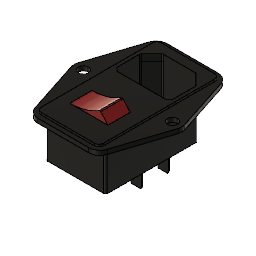
Controller PSU Assembly (Autodesk Fusion 360 archive; units mm, degrees)
design "IEC Inlet"
Autodesk Fusion 360 part; units mm, degrees
sketch "Sketch1" plane through (0, 0, 0) normal (0, 0, 1) x (1, 0, 0)
  line L0 (-25, 14) -> (25, 14)
  line L1 (27, 12) -> (27, -12)
  line L2 (25, -14) -> (-25, -14)
  line L3 (-27, -12) -> (-27, 12)
  arc A0 (-25, 14) -> (-27, 12) centre (-25, 12) ccw
  arc A1 (-27, -12) -> (-25, -14) centre (-25, -12) ccw
  arc A2 (25, -14) -> (27, -12) centre (25, -12) ccw
  arc A3 (27, 12) -> (25, 14) centre (25, 12) ccw
  dimension "d1" = 28
  dimension "d2" = 54
  dimension "d3" = 14
  dimension "d4" = 27
  dimension "d5" = 2
  constraint horizontal L0
  constraint vertical L1
  constraint horizontal L2
  constraint vertical L3
  constraint tangent L3 A0
  constraint tangent L0 A0
  constraint tangent L3 A1
  constraint tangent L2 A1
  constraint equal A0 A1
  constraint tangent L2 A2
  constraint tangent L1 A2
  constraint equal A0 A2
  constraint tangent L1 A3
  constraint tangent L0 A3
  constraint equal A0 A3
  measures "d1" distance of L0 L2
  measures "d2" distance of L1 L3
  measures "d3" distance of origin L2
  measures "d4" distance of origin L3
  measures "d5" radius of A0
extrude "Extrude1" add sketch "Sketch1" along normal blind 1
sketch "Sketch2" plane through (0, 0, 0) normal (0, 0, -1) x (1, 0, 0)
  arc A0 (27, 12) -> (25, 14) centre (25, 12) ccw
  line L0 (25, 14) -> (-25, 14)
  arc A1 (-25, 14) -> (-27, 12) centre (-25, 12) ccw
  line L1 (-27, 12) -> (-27, -12)
  arc A2 (-27, -12) -> (-25, -14) centre (-25, -12) ccw
  line L2 (-25, -14) -> (25, -14)
  arc A3 (25, -14) -> (27, -12) centre (25, -12) ccw
  line L3 (27, -12) -> (27, 12)
  line L4 (-29, 24.5) -> (29, 24.5)
  line L5 (29, 11.423) -> (29, -11.423)
  line L6 (29, -24.5) -> (-29, -24.5)
  line L7 (-29, -11.423) -> (-29, 11.423)
  circle A4 centre (0, -20) radius 2.25
  circle A5 centre (0, 20) radius 2.25
  line L8 (1.5487, -23.9955) -> (25.5487, -16.1771)
  line L9 (-1.5487, -23.9955) -> (-25.5487, -16.1771)
  line L10 (1.5487, 23.9955) -> (25.5487, 16.1771)
  line L11 (-1.5487, 23.9955) -> (-25.5487, 16.1771)
  arc A6 (25.5487, -16.1771) -> (29, -11.423) centre (24, -11.423) ccw
  arc A7 (29, 11.423) -> (25.5487, 16.1771) centre (24, 11.423) ccw
  arc A8 (-25.5487, 16.1771) -> (-29, 11.423) centre (-24, 11.423) ccw
  arc A9 (-29, -11.423) -> (-25.5487, -16.1771) centre (-24, -11.423) ccw
  arc A10 (-1.5487, -23.9955) -> (1.5487, -23.9955) centre (0, -19.2414) ccw
  arc A11 (1.5487, 23.9955) -> (-1.5487, 23.9955) centre (0, 19.2414) ccw
  point P0 (0, -24.5)
  point P1 (29, -15.0528)
  point P2 (-29, -15.0528)
  point P3 (0, 24.5)
  point P4 (29, 15.0528)
  point P5 (-29, 15.0528)
  dimension "d8" = 58
  dimension "d9" = 29
  dimension "d10" = 49
  dimension "d11" = 24.5
  dimension "d12" = 4.5
  dimension "d13" = 4.5
  dimension "d14" = 40
  dimension "d15" = 4.5
  dimension "d16" = 30.5
  dimension "d17" = 30.5
  dimension "d18" = 30.5
  dimension "d19" = 30.5
  dimension "d20" = 5
  dimension "d21" = 5
  constraint horizontal L4
  constraint vertical L5
  constraint horizontal L6
  constraint vertical L7
  constraint vertical origin A5.centre
  constraint vertical origin A4.centre
  constraint midpoint L6 P0
  constraint coincident L5 P1
  constraint coincident L7 P2
  constraint midpoint L4 P3
  constraint coincident L5 P4
  constraint coincident L7 P5
  constraint coincident P1 L8
  constraint coincident L6.start L5
  constraint tangent L8 A6
  constraint tangent L5 A6
  constraint coincident L4.end L5
  constraint coincident P4 L10
  constraint tangent L5 A7
  constraint tangent L10 A7
  constraint equal A6 A7
  constraint coincident P5 L11
  constraint coincident L4.start L7
  constraint tangent L11 A8
  constraint tangent L7 A8
  constraint equal A6 A8
  constraint coincident L6.end L7
  constraint coincident P2 L9
  constraint tangent L7 A9
  constraint tangent L9 A9
  constraint equal A6 A9
  constraint coincident P0 L9
  constraint coincident P0 L8
  constraint tangent L9 A10
  constraint tangent L8 A10
  constraint coincident P3 L10
  constraint coincident P3 L11
  constraint tangent L10 A11
  constraint tangent L11 A11
  constraint equal A10 A11
  measures "d8" distance of L5 L7
  measures "d9" distance of origin L7
  measures "d10" distance of L4 L6
  measures "d11" distance of origin L6
  measures "d12" diameter of A4
  measures "d13" diameter of A5
  measures "d14" distance of A4.centre A5.centre
  measures "d15" distance of L6 A4.centre
  measures "d16" distance of P0 P1
  measures "d17" distance of P0 P2
  measures "d18" distance of P3 P4
  measures "d19" distance of P3 P5
  measures "d20" radius of A6
  measures "d21" radius of A10
extrude "Extrude2" add sketch "Sketch2" along normal blind 2 contours A0 L0 A1 L1 A2 L2 A3 L3 | L5 L7 L8 L9 L10 L11 A6 A7 A8 A9 A10 A11
sketch "Sketch3" plane through (0, 0, -2) normal (0, 0, -1) x (1, 0, 0)
  circle A0 centre (0, 20) radius 2.25
  circle A1 centre (0, -20) radius 2.25
  arc A2 (29, 11.423) -> (25.5487, 16.1771) centre (24, 11.423) ccw
  line L0 (25.5487, 16.1771) -> (1.5487, 23.9955)
  arc A3 (1.5487, 23.9955) -> (-1.5487, 23.9955) centre (0, 19.2414) ccw
  line L1 (-1.5487, 23.9955) -> (-25.5487, 16.1771)
  arc A4 (-25.5487, 16.1771) -> (-29, 11.423) centre (-24, 11.423) ccw
  line L2 (-29, 11.423) -> (-29, -11.423)
  arc A5 (-29, -11.423) -> (-25.5487, -16.1771) centre (-24, -11.423) ccw
  line L3 (-25.5487, -16.1771) -> (-1.5487, -23.9955)
  arc A6 (-1.5487, -23.9955) -> (1.5487, -23.9955) centre (0, -19.2414) ccw
  line L4 (1.5487, -23.9955) -> (25.5487, -16.1771)
  arc A7 (25.5487, -16.1771) -> (29, -11.423) centre (24, -11.423) ccw
  line L5 (29, -11.423) -> (29, 11.423)
  line L6 (-22.5, 13.5) -> (22.5, 13.5)
  line L7 (23.5, 12.5) -> (23.5, -12.5)
  line L8 (22.5, -13.5) -> (-22.5, -13.5)
  line L9 (-23.5, -12.5) -> (-23.5, 12.5)
  arc A8 (23.5, 12.5) -> (22.5, 13.5) centre (22.5, 12.5) ccw
  arc A9 (22.5, -13.5) -> (23.5, -12.5) centre (22.5, -12.5) ccw
  arc A10 (-23.5, -12.5) -> (-22.5, -13.5) centre (-22.5, -12.5) ccw
  arc A11 (-22.5, 13.5) -> (-23.5, 12.5) centre (-22.5, 12.5) ccw
  dimension "d24" = 27
  dimension "d25" = 47
  dimension "d26" = 23.5
  dimension "d27" = 13.5
  dimension "d30" = 1
  constraint horizontal L6
  constraint vertical L7
  constraint horizontal L8
  constraint vertical L9
  constraint tangent L6 A8
  constraint tangent L7 A8
  constraint tangent L7 A9
  constraint tangent L8 A9
  constraint equal A8 A9
  constraint tangent L8 A10
  constraint tangent L9 A10
  constraint equal A8 A10
  constraint tangent L9 A11
  constraint tangent L6 A11
  constraint equal A8 A11
  measures "d24" distance of L6 L8
  measures "d25" distance of L7 L9
  measures "d26" distance of origin L9
  measures "d27" distance of origin L6
  measures "d30" radius of A8
extrude "Extrude3" add sketch "Sketch3" along normal blind 18 contours L6 L7 L8 L9 A8 A9 A10 A11
sketch "Sketch4" plane through (0, 0, -20) normal (0, 0, -1) x (1, 0, 0)
  arc A0 (23.5, 12.5) -> (22.5, 13.5) centre (22.5, 12.5) ccw
  line L0 (22.5, 13.5) -> (-22.5, 13.5)
  arc A1 (-22.5, 13.5) -> (-23.5, 12.5) centre (-22.5, 12.5) ccw
  line L1 (-23.5, 12.5) -> (-23.5, -12.5)
  arc A2 (-23.5, -12.5) -> (-22.5, -13.5) centre (-22.5, -12.5) ccw
  line L2 (-22.5, -13.5) -> (22.5, -13.5)
  arc A3 (22.5, -13.5) -> (23.5, -12.5) centre (22.5, -12.5) ccw
  line L3 (23.5, -12.5) -> (23.5, 12.5)
  line L4 (17.136, 13.5) -> (23.5, 7.136)
  line L5 (23.5, -7.136) -> (17.136, -13.5)
  dimension "d31" = 9
  dimension "d32" = 9
  dimension "d33" = 45
  dimension "d34" = 45
  constraint coincident L0 L4.start
  constraint coincident L3 L4.end
  constraint coincident L3 L5.start
  constraint coincident L2 L5.end
  measures "d31" distance of L5.start L5.end
  measures "d32" distance of L4.start L4.end
  measures "d33" angle of L3 L4
  measures "d34" angle of L3 L5
extrude "Extrude4" cut sketch "Sketch4" against normal blind 18 contours A0 L0 L3 L4 | L2 A3 L3 L5
sketch "Sketch5" plane through (0, 0, 1) normal (0, 0, 1) x (-1, 0, 0)
  arc A0 (-25, 14) -> (-27, 12) centre (-25, 12) ccw
  line L0 (-27, 12) -> (-27, -12)
  arc A1 (-27, -12) -> (-25, -14) centre (-25, -12) ccw
  line L1 (-25, -14) -> (25, -14)
  arc A2 (25, -14) -> (27, -12) centre (25, -12) ccw
  line L2 (27, -12) -> (27, 12)
  arc A3 (27, 12) -> (25, 14) centre (25, 12) ccw
  line L3 (25, 14) -> (-25, 14)
  line L4 (-8, -12.5) -> (-17.636, -12.5)
  line L5 (-23, -7.136) -> (-23, 7.136)
  line L6 (-17.636, 12.5) -> (-8, 12.5)
  line L7 (-6, 10.5) -> (-6, -10.5)
  line L8 (-18.3431, 12.2071) -> (-22.7071, 7.8431)
  line L9 (-22.7071, -7.8431) -> (-18.3431, -12.2071)
  arc A4 (-8, -12.5) -> (-6, -10.5) centre (-8, -10.5) ccw
  arc A5 (-6, 10.5) -> (-8, 12.5) centre (-8, 10.5) ccw
  arc A6 (-18.3431, -12.2071) -> (-17.636, -12.5) centre (-17.636, -11.5) ccw
  arc A7 (-23, -7.136) -> (-22.7071, -7.8431) centre (-22, -7.136) ccw
  arc A8 (-22.7071, 7.8431) -> (-23, 7.136) centre (-22, 7.136) ccw
  arc A9 (-17.636, 12.5) -> (-18.3431, 12.2071) centre (-17.636, 11.5) ccw
  point P0 (-18.0503, 12.5)
  point P1 (-23, 7.5503)
  point P2 (-23, -7.5503)
  point P3 (-18.0503, -12.5)
  dimension "d37" = 4
  dimension "d38" = 17
  dimension "d39" = 25
  dimension "d40" = 12.5
  dimension "d41" = 7
  dimension "d42" = 7
  dimension "d43" = 45
  dimension "d44" = 45
  dimension "d45" = 2
  dimension "d46" = 1
  constraint horizontal L4
  constraint vertical L5
  constraint horizontal L6
  constraint vertical L7
  constraint coincident L6 P0
  constraint coincident L5 P1
  constraint coincident L5 P2
  constraint coincident L4 P3
  constraint tangent L4 A4
  constraint tangent L7 A4
  constraint tangent L6 A5
  constraint tangent L7 A5
  constraint equal A4 A5
  constraint coincident P3 L9
  constraint tangent L4 A6
  constraint tangent L9 A6
  constraint coincident P2 L9
  constraint tangent L9 A7
  constraint tangent L5 A7
  constraint equal A6 A7
  constraint coincident P1 L8
  constraint tangent L5 A8
  constraint tangent L8 A8
  constraint equal A6 A8
  constraint coincident P0 L8
  constraint tangent L8 A9
  constraint tangent L6 A9
  constraint equal A6 A9
  measures "d37" distance of L0 L5
  measures "d38" distance of L5 L7
  measures "d39" distance of L4 L6
  measures "d40" distance of origin L6
  measures "d41" distance of P0 P1
  measures "d42" distance of P2 P3
  measures "d43" angle of L5 L9
  measures "d44" angle of L5 L8
  measures "d45" radius of A4
  measures "d46" radius of A6
extrude "Extrude5" cut sketch "Sketch5" against normal blind 18 contours L4 L5 L6 L7 L8 L9 A4 A5 A6 A7 A8 A9
sketch "Sketch6" plane through (0, 0, 1) normal (0, 0, 1) x (-1, 0, 0)
  line L0 (-17.636, 12.5) -> (-8, 12.5)
  arc A0 (-6, 10.5) -> (-8, 12.5) centre (-8, 10.5) ccw
  line L1 (-6, 10.5) -> (-6, -10.5)
  arc A1 (-8, -12.5) -> (-6, -10.5) centre (-8, -10.5) ccw
  line L2 (-8, -12.5) -> (-17.636, -12.5)
  arc A2 (-18.3431, -12.2071) -> (-17.636, -12.5) centre (-17.636, -11.5) ccw
  line L3 (-18.3431, -12.2071) -> (-22.7071, -7.8431)
  arc A3 (-23, -7.136) -> (-22.7071, -7.8431) centre (-22, -7.136) ccw
  line L4 (-23, -7.136) -> (-23, 7.136)
  arc A4 (-22.7071, 7.8431) -> (-23, 7.136) centre (-22, 7.136) ccw
  line L5 (-22.7071, 7.8431) -> (-18.3431, 12.2071)
  arc A5 (-17.636, 12.5) -> (-18.3431, 12.2071) centre (-17.636, 11.5) ccw
  arc A6 (-25, 14) -> (-27, 12) centre (-25, 12) ccw
  line L6 (-27, 12) -> (-27, -12)
  arc A7 (-27, -12) -> (-25, -14) centre (-25, -12) ccw
  line L7 (-25, -14) -> (25, -14)
  arc A8 (25, -14) -> (27, -12) centre (25, -12) ccw
  line L8 (27, -12) -> (27, 12)
  arc A9 (27, 12) -> (25, 14) centre (25, 12) ccw
  line L9 (25, 14) -> (-25, 14)
  line L10 (17, -8) -> (7, -8)
  line L11 (7, -8) -> (7, 8)
  line L12 (7, 8) -> (17, 8)
  line L13 (17, 8) -> (17, -8)
  line L14 (17, 4.5) -> (7, 4.5)
  dimension "d49" = 16
  dimension "d50" = 10
  dimension "d51" = 10
  dimension "d52" = 6
  dimension "d53" = 12.5
  constraint horizontal L10
  constraint vertical L11
  constraint horizontal L12
  constraint vertical L13
  constraint coincident L13 L14.start
  constraint coincident L11 L14.end
  constraint perpendicular L11 L14
  measures "d49" distance of L10 L12
  measures "d50" distance of L11 L13
  measures "d51" distance of L8 L13
  measures "d52" distance of L7 L10
  measures "d53" distance of L10 L14
extrude "Extrude6" add sketch "Sketch6" along normal blind 4 contours L11 L12 L13 L14
fillet "Fillet1" radius 25 1 edges at (-12, -4.5, 1)
sketch "Sketch7" plane through (-17, 0, 0) normal (-1, 0, 0) x (0, -1, 0)
  line L0 (-9.0647, 1) -> (8, 1)
  line L1 (8, 1) -> (8, 5)
  line L2 (8, 5) -> (4.5, 5)
  arc A0 (-9.0647, 1) -> (4.5, 5) centre (-9.0647, 26) ccw
  line L3 (4.5, 5) -> (8, 1)
  constraint coincident L2.end A0.end
  constraint coincident L0.end L1.start
extrude "Extrude7" cut sketch "Sketch7" against normal blind 10 contours L1 L2 L3
fillet "Fillet2" radius 0.5 1 edges at (-12, -4.5, 5)
sketch "Sketch9" plane through (0, 0, -20) normal (0, 0, -1) x (1, 0, 0)
  line L0 (23.5, 7.136) -> (17.136, 13.5)
  line L1 (17.136, 13.5) -> (-22.5, 13.5)
  arc A0 (-22.5, 13.5) -> (-23.5, 12.5) centre (-22.5, 12.5) ccw
  line L2 (-23.5, 12.5) -> (-23.5, -12.5)
  arc A1 (-23.5, -12.5) -> (-22.5, -13.5) centre (-22.5, -12.5) ccw
  line L3 (-22.5, -13.5) -> (17.136, -13.5)
  line L4 (17.136, -13.5) -> (23.5, -7.136)
  line L5 (23.5, -7.136) -> (23.5, 7.136)
  line L6 (-21.5, 12.5) -> (-8.5, 12.5)
  line L7 (-7.5, 11.5) -> (-7.5, -11.5)
  line L8 (-8.5, -12.5) -> (-21.5, -12.5)
  line L9 (-22.5, -11.5) -> (-22.5, 11.5)
  arc A2 (-21.5, 12.5) -> (-22.5, 11.5) centre (-21.5, 11.5) ccw
  arc A3 (-7.5, 11.5) -> (-8.5, 12.5) centre (-8.5, 11.5) ccw
  arc A4 (-8.5, -12.5) -> (-7.5, -11.5) centre (-8.5, -11.5) ccw
  arc A5 (-22.5, -11.5) -> (-21.5, -12.5) centre (-21.5, -11.5) ccw
  dimension "d62" = 1
  dimension "d63" = 1
  dimension "d64" = 1
  dimension "d65" = 15
  dimension "d66" = 1
  constraint horizontal L6
  constraint vertical L7
  constraint horizontal L8
  constraint vertical L9
  constraint tangent L6 A2
  constraint tangent L9 A2
  constraint tangent L6 A3
  constraint tangent L7 A3
  constraint equal A2 A3
  constraint tangent L7 A4
  constraint tangent L8 A4
  constraint equal A2 A4
  constraint tangent L8 A5
  constraint tangent L9 A5
  constraint equal A2 A5
  measures "d62" distance of L1 L6
  measures "d63" distance of L3 L8
  measures "d64" distance of L2 L9
  measures "d65" distance of L7 L9
  measures "d66" radius of A2
extrude "Extrude8" cut sketch "Sketch9" against normal blind 18 contours L6 L7 L8 L9 A2 A3 A4 A5
sketch "Sketch10" plane through (0, 0, -20) normal (0, 0, -1) x (1, 0, 0)
  line L0 (-22.5, -11.5) -> (-22.5, 11.5)
  arc A0 (-21.5, 12.5) -> (-22.5, 11.5) centre (-21.5, 11.5) ccw
  line L1 (-21.5, 12.5) -> (-8.5, 12.5)
  arc A1 (-7.5, 11.5) -> (-8.5, 12.5) centre (-8.5, 11.5) ccw
  line L2 (-7.5, 11.5) -> (-7.5, -11.5)
  arc A2 (-8.5, -12.5) -> (-7.5, -11.5) centre (-8.5, -11.5) ccw
  line L3 (-8.5, -12.5) -> (-21.5, -12.5)
  arc A3 (-22.5, -11.5) -> (-21.5, -12.5) centre (-21.5, -11.5) ccw
  line L4 (23.5, 7.136) -> (17.136, 13.5)
  line L5 (17.136, 13.5) -> (-22.5, 13.5)
  arc A4 (-22.5, 13.5) -> (-23.5, 12.5) centre (-22.5, 12.5) ccw
  line L6 (-23.5, 12.5) -> (-23.5, -12.5)
  arc A5 (-23.5, -12.5) -> (-22.5, -13.5) centre (-22.5, -12.5) ccw
  line L7 (-22.5, -13.5) -> (17.136, -13.5)
  line L8 (17.136, -13.5) -> (23.5, -7.136)
  line L9 (23.5, -7.136) -> (23.5, 7.136)
  line L10 (19.5, 2.5) -> (20, 2.5)
  line L11 (20, 2.5) -> (20, -2.5)
  line L12 (20, -2.5) -> (19.5, -2.5)
  line L13 (19.5, -2.5) -> (19.5, 2.5)
  line L14 (8.636, 9.5) -> (9.136, 9.5)
  line L15 (9.136, 9.5) -> (9.136, 4.5)
  line L16 (9.136, 4.5) -> (8.636, 4.5)
  line L17 (8.636, 4.5) -> (8.636, 9.5)
  line L18 (-3.364, 9.5) -> (-2.864, 9.5)
  line L19 (-2.864, 9.5) -> (-2.864, 4.5)
  line L20 (-2.864, 4.5) -> (-3.364, 4.5)
  line L21 (-3.364, 4.5) -> (-3.364, 9.5)
  dimension "d69" = 5
  dimension "d70" = 0.5
  dimension "d71" = 0.5
  dimension "d72" = 5
  dimension "d75" = 3.5
  dimension "d76" = 11
  dimension "d77" = 4
  dimension "d78" = 5
  dimension "d79" = 0.5
  dimension "d80" = 4
  dimension "d81" = 8
  dimension "d82" = 20
  constraint horizontal L10
  constraint vertical L11
  constraint horizontal L12
  constraint vertical L13
  constraint horizontal L14
  constraint vertical L15
  constraint horizontal L16
  constraint vertical L17
  constraint horizontal L18
  constraint vertical L19
  constraint horizontal L20
  constraint vertical L21
  measures "d69" distance of L10 L12
  measures "d70" distance of L11 L13
  measures "d71" distance of L15 L17
  measures "d72" distance of L14 L16
  measures "d75" distance of L9 L11
  measures "d76" distance of L7 L12
  measures "d77" distance of L5 L14
  measures "d78" distance of L18 L20
  measures "d79" distance of L19 L21
  measures "d80" distance of L5 L18
  measures "d81" distance of L4.end L15
  measures "d82" distance of L4.end L19
extrude "Extrude9" add sketch "Sketch10" along normal blind 10 contours L10 L11 L12 L13 | L14 L15 L16 L17 | L18 L19 L20 L21
sketch "Sketch11" plane through (-3.364, 0, 0) normal (-1, 0, 0) x (0, -1, 0)
  line L0 (9.5, -20) -> (4.5, -20)
  line L1 (4.5, -20) -> (4.5, -30)
  line L2 (4.5, -30) -> (9.5, -30)
  line L3 (9.5, -30) -> (9.5, -20)
  line L4 (5, -30) -> (4.5, -29.134)
  line L5 (9, -30) -> (9.5, -29.134)
  dimension "d85" = 1
  dimension "d86" = 1
  dimension "d87" = 30
  dimension "d88" = 30
  constraint coincident L2 L4.start
  constraint coincident L1 L4.end
  constraint coincident L2 L5.start
  constraint coincident L3 L5.end
  measures "d85" distance of L5.start L5.end
  measures "d86" distance of L4.start L4.end
  measures "d87" angle of L3 L5
  measures "d88" angle of L1 L4
extrude "Extrude10" cut sketch "Sketch11" against normal blind 15 contours L2 L3 L5 | L1 L2 L4
sketch "Sketch12" plane through (19.5, 0, 0) normal (-1, 0, 0) x (0, -1, 0)
  line L0 (2.5, -20) -> (-2.5, -20)
  line L1 (-2.5, -20) -> (-2.5, -30)
  line L2 (-2.5, -30) -> (2.5, -30)
  line L3 (2.5, -30) -> (2.5, -20)
  line L4 (2.5, -29.134) -> (2, -30)
  line L5 (-2, -30) -> (-2.5, -29.134)
  dimension "d91" = 1
  dimension "d92" = 1
  dimension "d93" = 30
  dimension "d94" = 30
  constraint coincident L3 L4.start
  constraint coincident L2 L4.end
  constraint coincident L2 L5.start
  constraint coincident L1 L5.end
  measures "d91" distance of L5.start L5.end
  measures "d92" distance of L4.start L4.end
  measures "d93" angle of L3 L4
  measures "d94" angle of L1 L5
extrude "Extrude11" cut sketch "Sketch12" against normal blind 0.5 contours L2 L3 L4 | L1 L2 L5
sketch "Sketch13" plane through (0, 0, -20) normal (0, 0, -1) x (1, 0, 0)
  line L0 (19.5, -2.5) -> (19.5, 2.5)
  line L1 (19.5, 2.5) -> (20, 2.5)
  line L2 (20, 2.5) -> (20, -2.5)
  line L3 (20, -2.5) -> (19.5, -2.5)
  line L4 (8.636, 4.5) -> (8.636, 9.5)
  line L5 (8.636, 9.5) -> (9.136, 9.5)
  line L6 (9.136, 9.5) -> (9.136, 4.5)
  line L7 (9.136, 4.5) -> (8.636, 4.5)
  line L8 (-3.364, 4.5) -> (-3.364, 9.5)
  line L9 (-3.364, 9.5) -> (-2.864, 9.5)
  line L10 (-2.864, 9.5) -> (-2.864, 4.5)
  line L11 (-2.864, 4.5) -> (-3.364, 4.5)
  line L12 (-22.5, -11.5) -> (-22.5, 11.5)
  arc A0 (-21.5, 12.5) -> (-22.5, 11.5) centre (-21.5, 11.5) ccw
  line L13 (-21.5, 12.5) -> (-8.5, 12.5)
  arc A1 (-7.5, 11.5) -> (-8.5, 12.5) centre (-8.5, 11.5) ccw
  line L14 (-7.5, 11.5) -> (-7.5, -11.5)
  arc A2 (-8.5, -12.5) -> (-7.5, -11.5) centre (-8.5, -11.5) ccw
  line L15 (-8.5, -12.5) -> (-21.5, -12.5)
  arc A3 (-22.5, -11.5) -> (-21.5, -12.5) centre (-21.5, -11.5) ccw
  line L16 (23.5, 7.136) -> (17.136, 13.5)
  line L17 (17.136, 13.5) -> (-22.5, 13.5)
  arc A4 (-22.5, 13.5) -> (-23.5, 12.5) centre (-22.5, 12.5) ccw
  line L18 (-23.5, 12.5) -> (-23.5, -12.5)
  arc A5 (-23.5, -12.5) -> (-22.5, -13.5) centre (-22.5, -12.5) ccw
  line L19 (-22.5, -13.5) -> (17.136, -13.5)
  line L20 (17.136, -13.5) -> (23.5, -7.136)
  line L21 (23.5, -7.136) -> (23.5, 7.136)
  line L22 (17.0773, 5.378) -> (22.5771, 5.378)
  line L23 (22.5771, 5.378) -> (22.5771, -4.9703)
  line L24 (22.5771, -4.9703) -> (17.0773, -4.9703)
  line L25 (17.0773, -4.9703) -> (17.0773, 5.378)
  constraint horizontal L22
  constraint vertical L23
  constraint horizontal L24
  constraint vertical L25
extrude "Extrude12" [suppressed]
equation "d3 = ( 28 / 2 ) * 1 mm"
equation "d4 = ( 54 / 2 ) * 1 mm"
equation "d9 = ( 58 / 2 ) * 1 mm"
equation "d11 = ( 49 / 2 ) * 1 mm"
equation "d26 = ( 47 / 2 ) * 1 mm"
equation "d27 = ( 27 / 2 ) * 1 mm"
equation "d40 = ( 25 / 2 ) * 1 mm"
equation "d76 = ( 27 / 2 ) * 1 mm - 2.5 mm"
